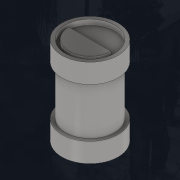
# Autodesk Inventor part: Middle handle
Saved by Autodesk Inventor 2021 (Build 250183000, 183)
## iProperties
Created: 2021-01-08
Part Number: Middle handle
Material: Generic
Document SubType Name: Modeling
Designer: Alex
Density: 1 g/cm^3
Appearance: Default
Author: Alex
Autodesk Inventor part; units mm, degrees
ref_plane "XZ Plane" through (0, 0, 0) normal (0, 1, 0) x (-1, 0, 0)
ref_plane "XY Plane" through (0, 0, 0) normal (0, 0, 1) x (1, 0, 0)
sketch "Sketch1" plane through (0, 0, 0) normal (0, 1, 0) x (-1, 0, 0)
  circle A0 centre (0, 0) radius 16
  circle A1 centre (0, 0) radius 14
  dimension "d0" = 32
  dimension "d1" = 28
  constraints: 2 centre point, 2 coincident
  measures "d0" diameter of A0
  measures "d1" diameter of A1
extrude "Extrusion1" add sketch "Sketch1" along normal blind 50 contours A1
sketch "Sketch2" plane through (0, 0, 0) normal (0, -1, 0) x (1, 0, 0)
  circle A0 centre (0, 0) radius 16
  dimension "d4" = 32
  constraints: 1 centre point, 1 coincident
  measures "d4" diameter of A0
extrude "Extrusion2" add sketch "Sketch2" against normal blind 11
sketch "Sketch3" plane through (0, 50, 0) normal (0, 1, 0) x (1, 0, 0)
  circle A0 centre (0, 0) radius 16
  constraints: 1 centre point, 1 coincident
extrude "Extrusion3" add sketch "Sketch3" against normal blind 11
ref_plane "Work Plane1" through (-14, 0, 0) normal (1, 0, 0) x (0, 1, 0)
sketch "Sketch5" plane through (-14, 0, 0) normal (1, 0, 0) x (0, 1, 0)
  line L0 (39, 14) -> (39, -14) construction
  line L1 (39, 0) -> (11, 0) construction
  line L2 (11, -14) -> (11, 14) construction
  line L3 (39, 0) -> (30, 0) construction
  line L4 (11, 0) -> (20, 0) construction
  circle A0 centre (30, 0) radius 3
  circle A1 centre (20, 0) radius 3
  point P0 (0, 0)
  dimension "d10" = 9
  dimension "d11" = 9
  dimension "d12" = 6
  dimension "d13" = 6
  constraints: 6 end point, 2 centre point, 2 coincident, 2 midpoint, 2 point on line
  measures "d10" distance of L1.start L3.end
  measures "d11" distance of L1.end L4.end
  measures "d12" diameter of A0
  measures "d13" diameter of A1
extrude "Extrusion4" cut sketch "Sketch5" along normal blind 8
sketch "Sketch6" plane through (-6, 30, 0) normal (-1, 0, 0) x (0, 0, 1)
  line L0 (-4.6081, 4.2685) -> (5.6465, 4.2685)
  line L1 (5.6465, 4.2685) -> (5.6465, -14.2936)
  line L2 (5.6465, -14.2936) -> (-4.6081, -14.2936)
  line L3 (-4.6081, -14.2936) -> (-4.6081, 4.2685)
  point P0 (0, -30)
  constraints: 8 end point, 2 parallel, 1 horizontal, 1 perpendicular
extrude "Extrusion5" add sketch "Sketch6" along normal blind 2
sketch "Sketch7" plane through (0, 50, 0) normal (0, 1, 0) x (1, 0, 0)
  circle A0 centre (0, 0) radius 14
  circle A1 centre (0, 0) radius 12
  dimension "d18" = 28
  dimension "d19" = 24
  constraints: 2 centre point, 2 coincident
  measures "d18" diameter of A0
  measures "d19" diameter of A1
extrude "Extrusion6" cut sketch "Sketch7" against normal blind 3
sketch "Sketch8" plane through (0, 50, 0) normal (0, 1, 0) x (1, 0, 0)
  circle A0 centre (0, 0) radius 12 projected
  line L0 (-12, 0) -> (12, 0)
  arc A1 (12, 0) -> (-12, 0) centre (0, 0) ccw
  constraints: 4 point on circle, 2 end point, 1 centre point, 1 coincident, 1 concentric, 1 horizontal
extrude "Extrusion7" cut sketch "Sketch8" against normal up to surface (3 mm away) contours L0 A0 picked at (2.994, 4.567)
sketch "Sketch9" plane through (0, 0, 0) normal (0, -1, 0) x (1, 0, 0)
  arc A0 (12, 0) -> (-12, 0) centre (0, 0) ccw projected
  line L0 (12, 0) -> (-12, 0) projected
  circle A1 centre (0, 0) radius 12
  circle A2 centre (0, 0) radius 14
  constraints: 2 coincident, 1 centre point, 1 horizontal alignment, 2 other
extrude "Extrusion8" cut sketch "Sketch9" against normal blind 3 contours L0 A0 | A1 L0 | A2
sketch "Sketch10" plane through (0, 3, 0) normal (0, -1, 0) x (1, 0, 0)
  line L0 (0, 0) -> (7, 0) construction
  line L1 (12, 0) -> (-12, 0) projected
  circle A0 centre (7, 0) radius 4
  constraints: 2 end point, 1 centre point, 1 coincident, 1 point on line
extrude "Extrusion9" cut sketch "Sketch10" against normal blind 3
body "Solid1"
